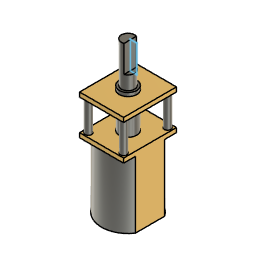
MicroMouse_Motor v2 (Autodesk Fusion 360 design; units mm, degrees)
Autodesk Fusion 360 part; units mm, degrees
note: some values were not read from the file. Set by a fixed rule: which sketch regions a step uses.
sketch "Sketch1" plane through (0, 0, 0) normal (0, 0, 1) x (1, 0, 0)
  circle A0 centre (0, 0) radius 6
  line L0 (-5, 6) -> (5, 6)
  line L1 (5, 6) -> (5, -6)
  line L2 (5, -6) -> (-5, -6)
  line L3 (-5, -6) -> (-5, 6)
  line L4 (-5, 6) -> (5, -6) construction
  line L5 (5, 6) -> (-5, -6) construction
  dimension "d1" = 12
  dimension "d2" = 10
  dimension "d3" = 12
  constraint coincident A0.centre origin
  constraint horizontal L0
  constraint perpendicular L0 L1
  constraint parallel L0 L2
  constraint parallel L1 L3
  constraint coincident L4 A0.centre
  constraint coincident L5 A0.centre
  measures "d1" diameter of A0
  measures "d2" distance of L1.end L2.end
  measures "d3" distance of L0.end L1.end
extrude "Extrude1" add sketch "Sketch1" along normal blind 15.1 contours A0 L1 L3
sketch "Sketch2" plane through (0, 0, 15.1) normal (0, 0, 1) x (-1, 0, 0)
  arc A0 (-5, -3.3166) -> (5, -3.3166) centre (0, 0) ccw
  line L0 (5, -3.3166) -> (5, 3.3166)
  arc A1 (5, 3.3166) -> (-5, 3.3166) centre (0, 0) ccw
  line L1 (-5, 3.3166) -> (-5, -3.3166)
  line L2 (5, -6) -> (-5, -6)
  line L3 (-5, -6) -> (-5, 6)
  line L4 (-5, 6) -> (5, 6)
  line L5 (5, 6) -> (5, -6)
  line L6 (5, -6) -> (-5, 6) construction
  line L7 (-5, -6) -> (5, 6) construction
  dimension "d6" = 10
  dimension "d7" = 12
  constraint horizontal L2
  constraint perpendicular L2 L3
  constraint parallel L2 L4
  constraint parallel L3 L5
  constraint coincident L6 A0.centre
  constraint coincident L7 A0.centre
  constraint coincident A0.centre A1.centre
  measures "d6" distance of L3.end L4.end
  measures "d7" distance of L2.end L3.end
extrude "Extrude2" add sketch "Sketch2" along normal blind 9
sketch "Sketch3" plane through (0, 0, 24.1) normal (0, 0, 1) x (-1, 0, 0)
  line L0 (5, 6) -> (-5, 6)
  line L1 (-5, 6) -> (-5, -6)
  line L2 (-5, -6) -> (5, -6)
  line L3 (5, -6) -> (5, 6)
  circle A0 centre (0, 0) radius 2
  circle A1 centre (0, 0) radius 1.5
  dimension "d10" = 4
  dimension "d11" = 3
  constraint coincident A0.centre A1.centre
  measures "d10" diameter of A0
  measures "d11" diameter of A1
extrude "Extrude3" add sketch "Sketch3" along normal blind 0.8 contours A0
extrude "Extrude4" add 1 faces at (-0.567, 0.5383, 24.1) along direction (0, 0, 1) blind 10
extrude "Extrude5" add sketch "Sketch3" along normal blind 10 contours A1
sketch "Sketch4" plane through (0, 0, 0) normal (0, 0, -1) x (1, 0, 0)
  arc A0 (-5, -3.3166) -> (5, -3.3166) centre (0, 0) ccw
  line L0 (5, -3.3166) -> (5, 3.3166)
  arc A1 (5, 3.3166) -> (-5, 3.3166) centre (0, 0) ccw
  line L1 (-5, 3.3166) -> (-5, -3.3166)
  circle A2 centre (0, 0) radius 2.5
  dimension "d18" = 5
  constraint concentric A0 A2
  measures "d18" diameter of A2
extrude "Extrude6" add sketch "Sketch4" along normal blind 1.2 contours A2
sketch "Sketch5" plane through (0, 0, 24.1) normal (0, 0, 1) x (-1, 0, 0)
  line L0 (-4, 5) -> (4, 5)
  line L1 (4, 5) -> (4, -5)
  line L2 (4, -5) -> (-4, -5)
  line L3 (-4, -5) -> (-4, 5)
  line L4 (-4, 5) -> (4, -5) construction
  line L5 (4, 5) -> (-4, -5) construction
  circle A0 centre (4, -5) radius 0.75
  circle A1 centre (-4, -5) radius 0.75
  circle A2 centre (4, 5) radius 0.75
  circle A3 centre (-4, 5) radius 0.75
  circle A4 centre (0, 0) radius 1.5
  dimension "d21" = 1.5
  dimension "d22" = 1.5
  dimension "d23" = 1.5
  dimension "d24" = 1.5
  dimension "d25" = 3
  constraint horizontal L0
  constraint perpendicular L0 L1
  constraint parallel L0 L2
  constraint parallel L1 L3
  constraint coincident L4 A4.centre
  constraint coincident L5 A4.centre
  constraint coincident A4.centre origin
  constraint coincident L1.end L2.start
  constraint coincident L2.end L3.start
  constraint coincident L0.end L1.start
  constraint coincident L0.start L3.end
  measures "d21" diameter of A0
  measures "d22" diameter of A1
  measures "d23" diameter of A2
  measures "d24" diameter of A3
  measures "d25" diameter of A4
extrude "Extrude7" cut 1 faces at (0.0498, 4.6648, 24.1) along direction (0, 0, -1) blind 7 from surface at 1
extrude "Extrude8" add sketch "Sketch5" against normal blind 8.5 contours L0 L3 A3 | L0 L3 A3 | L0 L1 A2 | L0 L1 A2 | L2 L3 A1 | L2 L3 A1 | L1 L2 A0 | L1 L2 A0 | A4
sketch "Sketch6" plane through (0, 0, 0) normal (0, 1, 0) x (1, 0, 0)
  line L0 (1, -28) -> (3, -28)
  line L1 (3, -28) -> (3, -35)
  line L2 (3, -35) -> (1, -35)
  line L3 (1, -35) -> (1, -28)
  constraint horizontal L0
  constraint vertical L1
  constraint horizontal L2
  constraint vertical L3
sketch "Sketch7" plane through (0, 0, 0) normal (0, 1, 0) x (1, 0, 0)
extrude "Extrude9" cut sketch "Sketch6" along normal blind 8
sketch "Sketch8" plane through (0, 0, 0) normal (0, 1, 0) x (1, 0, 0)
  line L0 (0.4932, -34.2266) -> (2, -34.2266)
  line L1 (2, -34.2266) -> (2, -28)
  line L2 (2, -28) -> (0.4932, -28)
  line L3 (0.4932, -28) -> (0.4932, -34.2266)
  constraint horizontal L0
  constraint vertical L1
  constraint horizontal L2
  constraint vertical L3
extrude "Extrude10" cut sketch "Sketch8" along normal blind 100
extrude "Extrude11" cut sketch "Sketch8" against normal blind 100
